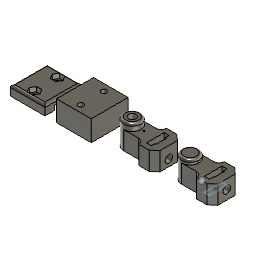
ThrustPlotter Parts (Autodesk Fusion 360 design; units mm, degrees)
Autodesk Fusion 360 part; units mm, degrees
box "BoxPrimitive1" add length 36 width 30 height 7 placed x (0, 1, 0) y (-1, 0, 0) z (0, 0, 1) at (30, 0, 0) makes body 1
sketch "Sketch2" plane through (30, 0, 0) normal (1, 0, 0) x (0, 1, 0)
  line L0 (0, 7) -> (0, 0)
  line L1 (0, 0) -> (36, 0)
  line L2 (36, 0) -> (36, 7)
  line L3 (36, 7) -> (0, 7)
  line L4 (25.5, -3.9) -> (10.5, -3.9)
  line L5 (10.5, -3.9) -> (10.5, 3.9)
  line L6 (10.5, 3.9) -> (25.5, 3.9)
  line L7 (25.5, 3.9) -> (25.5, -3.9)
  line L8 (25.5, -3.9) -> (10.5, 3.9) construction
  line L9 (10.5, -3.9) -> (25.5, 3.9) construction
  point P0 (18, 0)
  dimension "d8" = 15
  dimension "d9" = 7.8
  constraint horizontal L4
  constraint perpendicular L4 L5
  constraint parallel L4 L6
  constraint parallel L5 L7
  constraint coincident L8 P0
  constraint coincident L9 P0
  measures "d8" distance of L5.end L6.end
  measures "d9" distance of L4.end L5.end
extrude "Extrude1" cut sketch "Sketch2" against normal through all contours L1 L5 L6 L7 bodies 1
sketch "Sketch4" plane through (0, 0, 7) normal (0, 0, 1) x (-1, 0, 0)
  line L0 (-30, -36) -> (0, -36)
  line L1 (0, -36) -> (0, 0)
  line L2 (0, 0) -> (-30, 0)
  line L3 (-30, 0) -> (-30, -36)
  line L4 (-30, -10.5) -> (0, -10.5)
  line L5 (-15, -18) -> (-15, -8)
  line L6 (-15, -18) -> (-15, -28)
  circle A0 centre (-15, -8) radius 2.35
  circle A1 centre (-15, -28) radius 2.35
  line L7 (-19.6188, -27.9945) -> (-17.3142, -31.9972)
  line L8 (-17.3142, -31.9972) -> (-12.6954, -32.0028)
  line L9 (-12.6954, -32.0028) -> (-10.3812, -28.0055)
  line L10 (-10.3812, -28.0055) -> (-12.6858, -24.0028)
  line L11 (-12.6858, -24.0028) -> (-17.3046, -23.9972)
  line L12 (-17.3046, -23.9972) -> (-19.6188, -27.9945)
  line L13 (-19.6188, -7.9848) -> (-17.3225, -11.9924)
  line L14 (-17.3225, -11.9924) -> (-12.7037, -12.0076)
  line L15 (-12.7037, -12.0076) -> (-10.3812, -8.0152)
  line L16 (-10.3812, -8.0152) -> (-12.6775, -4.0076)
  line L17 (-12.6775, -4.0076) -> (-17.2963, -3.9924)
  line L18 (-17.2963, -3.9924) -> (-19.6188, -7.9848)
  point P0 (-15, -28)
  point P1 (-15, -8)
  dimension "d11" = 10
  dimension "d12" = 10
  dimension "d13" = 4.7
  dimension "d14" = 4.7
  dimension "d15" = 4
  dimension "d16" = 4
  constraint perpendicular L4 L5
  constraint parallel L5 L6
  constraint coincident P1 L5.end
  constraint coincident P0 L6.end
  measures "d11" distance of L5.start P1
  measures "d12" distance of L5.start P0
  measures "d13" diameter of A0
  measures "d14" diameter of A1
  measures "d15" distance of P0 L12
  measures "d16" distance of P1 L18
extrude "Extrude2" cut sketch "Sketch4" against normal through all contours A0 | A1 bodies 1
extrude "Extrude3" cut sketch "Sketch4" against normal blind 2.5 contours L4 L13 L15 L16 L17 L18 | L4 L5 L13 L14 | L4 L5 L14 L15 | L7 L8 L9 L10 L11 L12 bodies 1
extrude "Extrude4" cut 1 faces at (20, 0, 2.3333) along direction (0, 1, 0) blind 2 on bodies 1 bodies 1
extrude "Extrude5" cut 1 faces at (20, 36, 2.3333) along direction (0, -1, 0) blind 2 on bodies 1 bodies 1
extrude "Extrude6" add 1 faces at (25.7742, 15.9975, 7) along direction (0, 0, 1) blind 1.5 on bodies 1 bodies 1
fillet "Fillet1" radius 2 4 edges at (0, 18, 8.5) (15, 2, 8.5) (30, 18, 8.5) (15, 34, 8.5) on bodies 1
sketch "Sketch5" plane through (0, 0, 0) normal (0, 0, -1) x (1, 0, 0)
  line L0 (30, -2) -> (0, -2)
  line L1 (0, -2) -> (0, -10.5)
  line L2 (0, -10.5) -> (30, -10.5)
  line L3 (30, -10.5) -> (30, -2)
  circle A0 centre (15, -8) radius 2.35
  line L4 (0, -2) -> (30, -2)
  line L5 (30, -2) -> (30, -34)
  line L6 (30, -34) -> (0, -34)
  line L7 (0, -34) -> (0, -2)
  circle A1 centre (15, -8) radius 2.35
  circle A2 centre (15, -28) radius 2.35
  point P0 (30, -34)
  constraint horizontal L4
  constraint vertical L5
  constraint horizontal L6
  constraint vertical L7
  constraint coincident P0 L5.end
  constraint coincident L0.end L1.start
  constraint concentric A0 A1
extrude "Extrude7" add sketch "Sketch5" along normal blind 18 separate body makes body 2
sketch "Sketch6" plane through (0, 0, -18) normal (0, 0, -1) x (1, 0, 0)
  circle A0 centre (15, -28) radius 2.35
  circle A1 centre (15, -8) radius 2.35
  line L0 (0, -34) -> (30, -34)
  line L1 (30, -34) -> (30, -2)
  line L2 (30, -2) -> (0, -2)
  line L3 (0, -2) -> (0, -34)
move_body "Move1" bodies 2 to x (1, 0, 0) y (0, 1, 0) z (0, 0, 1) at (-110, 0, 0)
move_body "Move2" bodies 1 to x (1, 0, 0) y (0, 1, 0) z (0, 0, 1) at (-150, 0, 0)
move_body "Move3" bodies 2 to x (1, 0, 0) y (0, 1, 0) z (0, 0, 1) at (0, 0, 18)
sketch "Sketch7" plane through (0, 0, 0) normal (0, 0, 1) x (1, 0, 0)
  line L0 (10, 10) -> (14, 10)
  line L1 (14, 10) -> (14, 25)
  line L2 (14, 25) -> (10, 25)
  line L3 (10, 25) -> (10, 10)
  line L4 (16.5075, 5.5038) -> (7.5075, 5.5038)
  line L5 (7.5075, 5.5038) -> (7.5075, 29.5038)
  line L6 (7.5075, 29.5038) -> (16.5075, 29.5038)
  line L7 (16.5075, 29.5038) -> (16.5075, 5.5038)
  line L8 (16.5075, 5.5038) -> (7.5075, 29.5038) construction
  line L9 (7.5075, 5.5038) -> (16.5075, 29.5038) construction
  circle A0 centre (-10.0217, 17.5) radius 3.25
  circle A1 centre (-10.0217, 17.5) radius 7.5
  line L10 (10, 25) -> (-10.0217, 25)
  line L11 (10, 10) -> (-10.0217, 10)
  line L12 (14, 25) -> (21.5, 25)
  line L13 (21.5, 25) -> (21.5, 9.9336)
  line L14 (21.5, 9.9336) -> (14, 9.9336)
  line L15 (14, 9.9336) -> (14, 25)
  line L16 (15.0103, 22.0038) -> (9.0046, 22.0038)
  line L17 (9.0046, 22.0038) -> (9.0046, 13.0038)
  line L18 (9.0046, 13.0038) -> (15.0103, 13.0038)
  line L19 (15.0103, 13.0038) -> (15.0103, 22.0038)
  line L20 (15.0103, 22.0038) -> (9.0046, 13.0038) construction
  line L21 (9.0046, 22.0038) -> (15.0103, 13.0038) construction
  line L22 (16.5075, 29.5038) -> (21.5, 25)
  line L23 (16.5075, 5.5038) -> (21.5, 9.9336)
  point P0 (12.0075, 17.5038)
  point P1 (12.0075, 17.5038)
  dimension "d30" = 4
  dimension "d31" = 15
  dimension "d32" = 9
  dimension "d33" = 24
  dimension "d34" = 6.5
  dimension "d35" = 15
  dimension "d36" = 7.5
  dimension "d37" = 9
  constraint horizontal L0
  constraint vertical L1
  constraint horizontal L2
  constraint vertical L3
  constraint horizontal L4
  constraint perpendicular L4 L5
  constraint parallel L4 L6
  constraint parallel L5 L7
  constraint coincident L8 P1
  constraint coincident L9 P1
  constraint concentric A0 A1
  constraint coincident A1 L10.end
  constraint tangent A1 L10
  constraint coincident A1 L11.end
  constraint tangent A1 L11
  constraint parallel L10 L11
  constraint horizontal L12
  constraint vertical L13
  constraint horizontal L14
  constraint vertical L15
  constraint horizontal L16
  constraint perpendicular L16 L17
  constraint parallel L16 L18
  constraint parallel L17 L19
  constraint coincident L20 P1
  constraint coincident L21 P1
  constraint coincident P1 P0
  measures "d30" distance of L0.start L0.end
  measures "d31" distance of L0.start L2.end
  measures "d32" distance of L5.end L6.end
  measures "d33" distance of L4.end L5.end
  measures "d34" diameter of A0
  measures "d35" diameter of A1
  measures "d36" distance of L1.end L12.end
  measures "d37" distance of L16.end L17.end
extrude "Extrude9" add sketch "Sketch7" along normal blind 20 separate body contours L3 L5 L10 L11 L16 L17 L18 | L0 L4 L5 L7 L11 L14 L15 | L1 L7 L12 L14 L15 L16 L18 L19 | L3 L16 L17 L18 | L5 A1 L10 L11 | L2 L5 L6 L7 L10 L12 | L7 L14 L23 | L7 L12 L13 L14 | L7 L12 L22 makes body 3
extrude "Extrude10" add sketch "Sketch7" along normal blind 26 contours A1 bodies 3
fillet "Fillet2" radius 2 1 edges at (-17.0142, 14.7879, 26) on bodies 3
fillet "Fillet3" radius 4.5 2 edges at (7.5075, 10, 10) (7.5075, 25, 10) on bodies 3
sketch "Sketch8" plane through (21.5, 0, 0) normal (1, 0, 0) x (0, 1, 0)
  line L0 (9.9336, 0) -> (25, 0)
  line L1 (25, 0) -> (25, 20)
  line L2 (25, 20) -> (9.9336, 20)
  line L3 (9.9336, 20) -> (9.9336, 0)
  circle A0 centre (17.5, 10) radius 3.225
  dimension "d48" = 6.45
  measures "d48" diameter of A0
extrude "Extrude11" cut sketch "Sketch8" against normal blind 7 contours A0 bodies 3
sketch "Sketch9" plane through (0, 0, 0) normal (0, 0, 1) x (1, 0, 0)
  circle A0 centre (-10.0217, 17.5) radius 7.5
  line L0 (7.5075, 29.5038) -> (16.5075, 29.5038)
  line L1 (16.5075, 29.5038) -> (16.5075, 5.5038)
  line L2 (16.5075, 5.5038) -> (7.5075, 5.5038)
  line L3 (7.5075, 5.5038) -> (7.5075, 29.5038)
  line L4 (14.1325, 9.8788) -> (9.8825, 9.8788)
  line L5 (9.8825, 9.8788) -> (9.8825, 25.1288)
  line L6 (9.8825, 25.1288) -> (14.1325, 25.1288)
  line L7 (14.1325, 25.1288) -> (14.1325, 9.8788)
  line L8 (14.1325, 9.8788) -> (9.8825, 25.1288) construction
  line L9 (9.8825, 9.8788) -> (14.1325, 25.1288) construction
  line L10 (16.5075, 29.5038) -> (21.5, 25)
  line L11 (16.5075, 29.5038) -> (21.5, 25)
  line L12 (21.5, 9.9336) -> (21.5, 25)
  line L13 (21.5, 9.9336) -> (16.5075, 5.5038)
  line L14 (7.5075, 25) -> (-10.0217, 25)
  line L15 (7.5075, 10) -> (-10.0217, 10)
  circle A1 centre (-10.0217, 17.5) radius 1
  line L16 (9.1325, 22.0038) -> (14.8825, 22.0038)
  line L17 (14.8825, 22.0038) -> (14.8825, 13.0038)
  line L18 (14.8825, 13.0038) -> (9.1325, 13.0038)
  line L19 (9.1325, 13.0038) -> (9.1325, 22.0038)
  line L20 (9.1325, 22.0038) -> (14.8825, 13.0038) construction
  line L21 (14.8825, 22.0038) -> (9.1325, 13.0038) construction
  point P0 (-10.0217, 17.5)
  point P1 (7.5075, 29.5038)
  point P2 (16.5075, 5.5038)
  point P3 (12.0075, 17.5038)
  point P4 (12.0075, 17.5038)
  point P5 (21.5, 25)
  point P6 (21.5, 9.9336)
  point P7 (-10.0217, 25)
  point P8 (-10.0217, 10)
  point P9 (12.0075, 17.5038)
  dimension "d51" = 4.25
  dimension "d52" = 15.25
  dimension "d53" = 2
  dimension "d67" = 5.75
  dimension "d68" = 9
  constraint coincident P0 A0.centre
  constraint horizontal L0
  constraint vertical L1
  constraint horizontal L2
  constraint vertical L3
  constraint coincident P2 L1.end
  constraint coincident P1 L0.start
  constraint horizontal L4
  constraint perpendicular L4 L5
  constraint parallel L4 L6
  constraint parallel L5 L7
  constraint coincident L8 P9
  constraint coincident L9 P9
  constraint coincident P9 P4
  constraint coincident P5 L10.end
  constraint coincident P6 L12.start
  constraint coincident L3 L14.start
  constraint coincident P7 L14.end
  constraint tangent A0 L14
  constraint coincident L3 L15.start
  constraint coincident P8 L15.end
  constraint tangent A0 L15
  constraint horizontal L16
  constraint perpendicular L16 L17
  constraint parallel L16 L18
  constraint parallel L17 L19
  constraint coincident L20 P9
  constraint coincident L21 P9
  measures "d51" distance of L5.end L6.end
  measures "d52" distance of L4.end L5.end
  measures "d53" diameter of A1
  measures "d67" distance of L17.end L18.end
  measures "d68" distance of L16.end L17.end
extrude "Extrude12" add sketch "Sketch9" along normal blind 16 separate body contours A0 L3 L14 L15 | L0 L1 L2 L3 | L1 L10 L11 L12 L13 | L5 L16 L18 L19 makes body 4
extrude "Extrude13" add sketch "Sketch9" along normal blind 20 contours A0 bodies 4
sketch "Sketch10" plane through (0, 0, 20) normal (0, 0, 1) x (-1, 0, 0)
  circle A0 centre (10.0217, -17.5) radius 1
  circle A1 centre (10.0217, -17.5) radius 7.5
  circle A2 centre (10.0217, -17.5) radius 1
  constraint concentric A0 A2
extrude "Extrude14" add sketch "Sketch10" against normal blind 2 contours A0 A2 bodies 4
fillet "Fillet4" radius 2 1 edges at (-17.0142, 14.7879, 20) on bodies 4
fillet "Fillet5" radius 4.5 2 edges at (7.5075, 10, 8) (7.5075, 25, 8) on bodies 4
sketch "Sketch11" plane through (21.5, 0, 0) normal (1, 0, 0) x (0, 1, 0)
  line L0 (9.9336, 0) -> (25, 0)
  line L1 (25, 0) -> (25, 16)
  line L2 (25, 16) -> (9.9336, 16)
  line L3 (9.9336, 16) -> (9.9336, 0)
  circle A0 centre (17.5, 8) radius 3.225
  dimension "d64" = 6.45
  measures "d64" diameter of A0
extrude "Extrude15" cut sketch "Sketch11" against normal blind 8 contours A0 bodies 4
extrude "Extrude16" cut 1 faces at (-0.2493, 17.5, 0) along direction (0, 0, 1) blind 4 on bodies 3 bodies 3
sketch "Sketch12" plane through (0, 0, 4) normal (0, 0, -1) x (1, 0, 0)
  circle A0 centre (-10.0217, -17.5) radius 3.25
  line L0 (15.0103, -13.0038) -> (15.0103, -22.0038)
  line L1 (15.0103, -22.0038) -> (14, -22.0038)
  line L2 (14, -22.0038) -> (14, -25)
  line L3 (14, -25) -> (10, -25)
  line L4 (10, -25) -> (10, -10)
  line L5 (10, -10) -> (14, -10)
  line L6 (14, -10) -> (14, -13.0038)
  line L7 (14, -13.0038) -> (15.0103, -13.0038)
  line L8 (16.5075, -5.5038) -> (7.5075, -5.5038)
  arc A1 (3.0075, -10) -> (7.5075, -5.5038) centre (3.0075, -5.5) ccw
  line L9 (3.0075, -10) -> (-10.0217, -10)
  arc A2 (-10.0217, -10) -> (-10.0217, -25) centre (-10.0217, -17.5) ccw
  line L10 (-10.0217, -25) -> (3.0075, -25)
  arc A3 (7.5075, -29.5) -> (3.0075, -25) centre (3.0075, -29.5) ccw
  line L11 (7.5075, -29.5) -> (7.5075, -29.5038)
  line L12 (7.5075, -29.5038) -> (16.5075, -29.5038)
  line L13 (16.5075, -29.5038) -> (21.5, -25)
  line L14 (21.5, -25) -> (21.5, -9.9336)
  line L15 (21.5, -9.9336) -> (16.5075, -5.5038)
  line L16 (14.125, -25.125) -> (9.875, -25.125)
  line L17 (9.875, -25.125) -> (9.875, -9.875)
  line L18 (9.875, -9.875) -> (14.125, -9.875)
  line L19 (14.125, -9.875) -> (14.125, -25.125)
  line L20 (14.125, -25.125) -> (9.875, -9.875) construction
  line L21 (9.875, -25.125) -> (14.125, -9.875) construction
  circle A4 centre (0, -17.5) radius 0.75
  point P0 (12, -17.5)
  dimension "d71" = 4.25
  dimension "d72" = 15.25
  dimension "d74" = 1.5
  constraint horizontal L16
  constraint perpendicular L16 L17
  constraint parallel L16 L18
  constraint parallel L17 L19
  constraint coincident L20 P0
  constraint coincident L21 P0
  measures "d71" distance of L17.end L18.end
  measures "d72" distance of L16.end L17.end
  measures "d74" diameter of A4
extrude "Extrude17" cut sketch "Sketch12" against normal through all contours L1 L2 L3 L4 L5 L6 L7 L16 L17 L18 L19 bodies 3
extrude "Extrude18" cut sketch "Sketch12" against normal through all contours A4 bodies 3
move_body "Move4" bodies 3 to x (1, 0, 0) y (0, 1, 0) z (0, 0, 1) at (-50, 0, -4)
named bodies: "ThrustPlotter Clamp", "ThrustPlotter Spacer", "ThrustPlotter Nose", "ThrustPlotter Tail"
